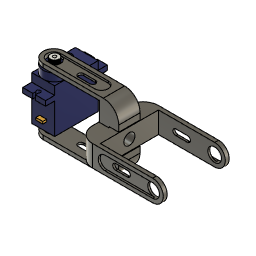
Part_1 v2 (Autodesk Fusion 360 design; units mm, degrees)
Autodesk Fusion 360 part; units mm, degrees
sketch "Left" plane through (0, 0, 0) normal (1, 0, 0) x (0, 0, -1) in component "_Servo-90.427e8e22-afa0-40e2-88ac-6b67eb2e57ee v1"
  line L0 (-21.4055, -22.0984) -> (1.0945, -22.0984)
  line L1 (-21.4055, 4.6016) -> (1.0945, 4.6016)
  line L2 (-21.4055, 0.6016) -> (1.0945, 0.6016)
  line L3 (-21.4055, 0.6016) -> (-21.4055, 4.6016)
  line L4 (5.7945, -22.0984) -> (5.7945, -6.1984)
  line L5 (-26.1055, -6.1984) -> (-26.1055, -3.6984)
  line L6 (-26.1055, -3.6984) -> (-21.4055, -3.6984)
  line L7 (1.0945, -3.6984) -> (5.7945, -3.6984)
  line L8 (-26.1055, -6.1984) -> (-21.4055, -6.1984)
  line L9 (1.0945, -6.1984) -> (5.7945, -6.1984)
  line L10 (1.0945, -22.0984) -> (1.0945, -6.1984)
  line L11 (1.0945, -3.6984) -> (1.0945, 0.6016)
  line L12 (-21.4055, -22.0984) -> (-21.4055, -6.1984)
  line L13 (-21.4055, -3.6984) -> (-21.4055, 0.6016)
  line L14 (-15.5055, 0.6016) -> (-15.5055, 13)
  line L15 (-6.7055, 0.6016) -> (-6.7055, 13)
  line L16 (1.0945, -22.0984) -> (1.0945, -6.1984)
  line L17 (1.0945, -3.6984) -> (1.0945, 13)
  line L18 (5.7945, -3.6984) -> (5.7945, -6.1984)
  dimension "d1" = 22.5
  dimension "d2" = 26.7
  dimension "d3" = 22.7
  dimension "d4" = 4
  dimension "d5" = 22.7
  dimension "d13" = 5.9
  constraint perpendicular L1 L3
  constraint parallel L0 L6
  constraint parallel L0 L8
  constraint parallel L5 L12
  constraint coincident L6.end L12
  constraint coincident L7.start L10
  constraint collinear L6 L7
  constraint collinear L8 L9
  constraint parallel L4 L10
  constraint collinear L10 L11
  constraint collinear L12 L13
  constraint parallel L3 L14
  constraint parallel L14 L16
  constraint collinear L16 L17
  constraint parallel L14 L15
  constraint coincident L2 L15.start
  constraint coincident L2 L14.start
  constraint perpendicular L9 L18
  measures "d1" distance of L0.start L0.end
  measures "d4" distance of L1.start L2.start
  measures "d5" distance of L0.start L2.start
  measures "d13" distance of L3 L14
extrude "Extrude1" add sketch "Left" along normal mid plane 11.8 contours L0 L2 L5 L6 L7 L8 L9 L10 L11 L12 L13 L16 L17 L18 makes body 1 in component "_Servo-90.427e8e22-afa0-40e2-88ac-6b67eb2e57ee v1"
sketch "TOP" plane through (0, 0.6016, 0) normal (0, 1, 0) x (-1, 0, 0) in component "_Servo-90.427e8e22-afa0-40e2-88ac-6b67eb2e57ee v1"
  line L0 (5.9, 21.4055) -> (-5.9, 21.4055)
  line L1 (-5.9, 21.4055) -> (-5.9, -1.0945)
  line L2 (-5.9, -1.0945) -> (5.9, -1.0945)
  line L3 (5.9, -1.0945) -> (5.9, 21.4055)
  circle A0 centre (0, 15.5055) radius 2.3
  circle A1 centre (0, 15.5055) radius 0.85
  line L4 (0, -1.0945) -> (0, 27)
  line L5 (0, 27) -> (0, -1.0945)
  arc A2 (-2.5, 9.2055) -> (2.5, 9.2055) centre (0, 9.2055) ccw
  line L6 (-2.5, 9.2055) -> (-2.5, 10.1613)
  line L7 (2.5, 9.2055) -> (2.5, 10.1613)
  arc A3 (2.5, 10.1613) -> (-2.5, 10.1613) centre (0, 15.5055) ccw
  line L8 (5.9, -5.7945) -> (-5.9, -5.7945)
  line L9 (-0.65, -4.2545) -> (-0.65, -5.7945)
  line L10 (0.65, -4.2545) -> (0.65, -5.7945)
  arc A4 (0.65, -4.2545) -> (-0.65, -4.2545) centre (0, -3.4945) ccw
  line L11 (5.9, 26.1055) -> (-5.9, 26.1055)
  arc A5 (-0.65, 24.5654) -> (0.65, 24.5654) centre (0, 23.8055) ccw
  line L12 (0.65, 24.5654) -> (0.65, 26.1055)
  line L13 (-0.65, 24.5654) -> (-0.65, 26.1055)
  point P0 (0, 15.5055)
  point P1 (0, 6.7055)
  point P2 (0, -1.0945)
  point P3 (5.9, -5.7945)
  point P4 (-5.9, -5.7945)
  point P5 (0, -5.7945)
  point P6 (5.9, 26.1055)
  point P7 (-5.9, 26.1055)
  point P8 (0, 26.1055)
  point P9 (0, 21.4055)
  dimension "d16" = 4.6
  dimension "d17" = 1.7
  dimension "d18" = 11.8
  dimension "d27" = 2
  dimension "d31" = 2
  constraint coincident P0 A0.centre
  constraint concentric A1 A3
  constraint coincident P1 A2
  constraint coincident P2 L4.start
  constraint perpendicular L0 L4
  constraint parallel L4 L6
  constraint parallel L4 L7
  constraint coincident P3 L8.start
  constraint coincident P4 L8.end
  constraint coincident P6 L11.start
  constraint coincident P7 L11.end
  constraint coincident L11 L12.end
  constraint coincident L11 L13.end
  measures "d16" diameter of A0
  measures "d17" diameter of A1
  measures "d18" diameter of A3
  measures "d27" diameter of A4
  measures "d31" diameter of A5
extrude "Extrude2" add sketch "TOP" along normal blind 4 contours A0 L4 L5 A2 L7 A3 | A0 L4 L5 A2 L6 A3 bodies 1 in component "_Servo-90.427e8e22-afa0-40e2-88ac-6b67eb2e57ee v1"
extrude "Extrude3" add sketch "TOP" along normal blind 7.2 separate body contours A0 A1 L4 L5 | A0 A1 L4 L5 makes body 2 in component "_Servo-90.427e8e22-afa0-40e2-88ac-6b67eb2e57ee v1"
extrude "Extrude4" cut sketch "TOP" against normal through all contours L4 L5 L11 A5 L13 | L4 L5 L11 A5 L12 bodies 1 in component "_Servo-90.427e8e22-afa0-40e2-88ac-6b67eb2e57ee v1"
extrude "Extrude5" cut sketch "TOP" against normal through all contours L8 L9 L10 A4 bodies 1 in component "_Servo-90.427e8e22-afa0-40e2-88ac-6b67eb2e57ee v1"
sketch "Front" plane through (0, 0, 21.4055) normal (0, 0, 1) x (1, 0, 0) in component "_Servo-90.427e8e22-afa0-40e2-88ac-6b67eb2e57ee v1"
  line L0 (-5.9, -22.0984) -> (5.9, -22.0984)
  line L1 (5.9, -22.0984) -> (5.9, -6.1984)
  line L2 (5.9, -6.1984) -> (-5.9, -6.1984)
  line L3 (-5.9, -6.1984) -> (-5.9, -22.0984)
  line L4 (-1.8, -17.5984) -> (1.8, -17.5984)
  line L5 (0, -22.0984) -> (0, -6.1984)
  line L6 (1.8, -17.5984) -> (1.8, -16.3984)
  line L7 (-1.8, -17.5984) -> (-1.8, -16.3984)
  line L8 (-1.8, -16.3984) -> (1.8, -16.3984)
extrude "Extrude6" add sketch "Front" along normal blind 2 separate body contours L4 L5 L6 L8 | L4 L5 L7 L8 makes body 3 in component "_Servo-90.427e8e22-afa0-40e2-88ac-6b67eb2e57ee v1"
copy_body "Body->Comp1" bodies 3 removing the originals makes body 4 in component "Prikljiček"
copy_body "Body->Comp2" bodies 2 removing the originals makes body 5 in component "OSovina"
copy_body "Body->Comp3" bodies 1 removing the originals makes body 6 in component "Ohisje"
sketch "Sketch1" plane through (0, 7.8016, 0) normal (0, 1, 0) x (-1, 0, 0) in component "OSovina"
  circle A0 centre (0, 15.5055) radius 0.85
  circle A1 centre (0, 15.5055) radius 2.3
  circle A2 centre (0, 15.5055) radius 2.3
  circle A3 centre (-0.0134, 13.2055) radius 0.125
  dimension "d42" = 0.25
  constraint coincident A2 A3.centre
  measures "d42" diameter of A3
extrude "Extrude1'" cut sketch "Sketch1" against normal up to surface (3.2 mm away) contours A1 A2 A3 | A1 A2 A3 picked at (-0.0101, 13.2473) picked at (-0.0141, 13.1641) bodies 5 in component "OSovina"
pattern_circular "C-Pattern1" count 28 over 360 about axis through (0, 15.4797, 15.5055) along (0, -1, 0) of "Extrude1'" in component "OSovina"
move_body "Move1" bodies 5 to x (1, 0, 0) y (0, 0, 1) z (0, -1, 0) at (0, 5.4071, 22.4039) in component "OSovina"
move_body "Move1'" bodies 6 to x (1, 0, 0) y (0, 0, 1) z (0, -1, 0) at (0, 5.4071, 22.4039) in component "Ohisje"
move_body "Move1''" bodies 4 to x (1, 0, 0) y (0, 0, 1) z (0, -1, 0) at (0, 5.4071, 22.4039) in component "Prikljiček"
sketch "Part_1" plane through (0, 0, 0) normal (0, 0, 1) x (1, 0, 0)
  line L0 (45, -13) -> (20, -13)
  line L1 (20, -2) -> (45, -2)
  line L2 (45, -2) -> (45, -13)
  arc A0 (20, -2) -> (20, -13) centre (20, -7.5) ccw
  circle A1 centre (20, -7.5) radius 3.5
  line L3 (45, -2) -> (59, -2)
  line L4 (59, -13) -> (45, -13)
  line L5 (45, -13) -> (45, -2)
  line L6 (59, -2) -> (59, -13)
  line L7 (20, -4) -> (43, -4)
  line L8 (43, -4) -> (43, -11)
  line L9 (43, -11) -> (20, -11)
  line L10 (40, -6) -> (34, -6)
  line L11 (40, -9) -> (33.9861, -9.0001)
  arc A2 (34, -6) -> (33.9861, -9.0001) centre (33.9861, -7.5) ccw
  arc A3 (40, -9) -> (40, -6) centre (40.068, -7.5) ccw
  constraint horizontal L0
  constraint horizontal L1
  constraint vertical L2
  constraint tangent L0 A0
  constraint horizontal L3
  constraint horizontal L4
  constraint vertical L5
  constraint coincident A1 L7.start
  constraint tangent A1 L7
  constraint horizontal L7
  constraint perpendicular L7 L8
  constraint coincident A1 L9.end
  constraint tangent A1 L9
  constraint perpendicular L8 L9
  constraint perpendicular L8 L10
  constraint tangent L11 A2
extrude "Extrude1''" add sketch "Part_1" along normal blind 30 and the other way blind 4 separate body contours L0 L1 L2 A0 L5 | L2 L3 L4 L5 L6 | A1 L7 L8 L9 makes body 7
sketch "Cut_1" plane through (0, -13, 0) normal (0, -1, 0) x (1, 0, 0)
  line L0 (59, -4) -> (59, 30)
  line L1 (59, 30) -> (20, 30)
  line L2 (20, -4) -> (59, -4)
  line L3 (49, 13) -> (49, 28)
  line L4 (49, 28) -> (13, 28)
  line L5 (13, 28) -> (13, 13)
  line L6 (49, 13) -> (49, -2)
  line L7 (49, -2) -> (13, -2)
  line L8 (13, -2) -> (13, 13)
  line L9 (59, 13) -> (59, 18.5)
  line L10 (59, 13) -> (59, 7.5)
  line L11 (54, 7.5) -> (54, 18.5)
  line L12 (59, 18.5) -> (59, 18.8)
  line L13 (59, 18.8) -> (54, 18.8)
  line L14 (54, 18.8) -> (54, 18.5)
  line L15 (59, 7.5) -> (59, 7.2)
  line L16 (59, 7.2) -> (54, 7.2)
  line L17 (54, 7.2) -> (54, 7.5)
  dimension "d10" = 34
  dimension "d19" = 10
  dimension "d21" = 17
  dimension "d26" = 5.5
  dimension "d28" = 5.5
  dimension "d29" = 5
  dimension "d30" = 11
  dimension "d36" = 0.3
  dimension "d37" = 0.3
  constraint vertical L3
  constraint horizontal L4
  constraint vertical L5
  constraint vertical L6
  constraint horizontal L7
  constraint vertical L8
  constraint parallel L0 L9
  constraint perpendicular L1 L10
  constraint vertical L12
  constraint horizontal L13
  constraint vertical L14
  constraint vertical L15
  constraint horizontal L16
  constraint vertical L17
  measures "d10" distance of L0.start L0.end
  measures "d19" distance of L0 L3.end
  measures "d21" distance of L0.start L9.start
  measures "d26" distance of L9.start L9.end
  measures "d28" distance of L9.start L10.end
  measures "d29" distance of L10.end L11.start
  measures "d30" distance of L11.start L11.end
  measures "d36" distance of L9.end L12.end
  measures "d37" distance of L10.end L15.end
extrude "Extrude2'" cut sketch "Cut_1" against normal blind 16 contours L3 L4 L5 L6 L7 L8 bodies 7
extrude "Extrude3'" cut sketch "Cut_1" against normal blind 16 contours L0 L9 L10 L11 L12 L13 L14 L15 L16 L17 bodies 7
fillet "Fillet1" radius 8 2 edges at (59, -7.5, 30) (59, -7.5, -4) on bodies 7
sketch "Cut_2" plane through (0, 0, 30) normal (0, 0, 1) x (-1, 0, 0)
  line L0 (-51, 13) -> (-51, 2)
  line L1 (-51, 2) -> (-20, 2)
  arc A0 (-20, 2) -> (-20, 13) centre (-20, 7.5) ccw
  line L2 (-20, 13) -> (-51, 13)
  arc A1 (-40, 9) -> (-40, 6) centre (-40.068, 7.5) ccw
  line L3 (-40, 9) -> (-33.9861, 9.0001)
  arc A2 (-34, 6) -> (-33.9861, 9.0001) centre (-33.9861, 7.5) ccw
  line L4 (-34, 6) -> (-40, 6)
  circle A3 centre (-20, 7.5) radius 3.5
  line L5 (-20, 4) -> (-44.5538, 4)
  line L6 (-20, 11) -> (-44.5538, 11)
  arc A4 (-44.5538, 11) -> (-44.5538, 4) centre (-44.5538, 7.5) ccw
  dimension "d51" = 24.5538
  dimension "d53" = 7
  constraint coincident A3 L5.start
  constraint coincident A3 L6.start
  constraint tangent L6 A4
  measures "d51" distance of A0.centre A4.centre
  measures "d53" distance of L5.end L6.end
extrude "Extrude4'" cut sketch "Cut_2" against normal blind 1 contours A3 L5 L6 A4 bodies 7
sketch "Cut_3" plane through (0, 0, -4) normal (0, 0, -1) x (1, 0, 0)
  line L0 (51, 2) -> (51, 13)
  line L1 (51, 13) -> (20, 13)
  arc A0 (20, 13) -> (20, 2) centre (20, 7.5) ccw
  line L2 (20, 2) -> (51, 2)
  circle A1 centre (20, 7.5) radius 3.5
  arc A2 (40, 6) -> (40, 9) centre (40.068, 7.5) ccw
  line L3 (40, 6) -> (34, 6)
  arc A3 (33.9861, 9.0001) -> (34, 6) centre (33.9861, 7.5) ccw
  line L4 (33.9861, 9.0001) -> (40, 9)
  line L5 (20, 11) -> (44.5538, 11)
  line L6 (20, 4) -> (44.5538, 4)
  arc A4 (44.5538, 4) -> (44.5538, 11) centre (44.5538, 7.5) ccw
  dimension "d52" = 24.5538
  dimension "d54" = 7
  constraint coincident A1 L5.start
  constraint tangent L5 A4
  constraint coincident A1 L6.start
  constraint tangent L6 A4
  measures "d52" distance of A0.centre A4.centre
  measures "d54" diameter of A4
extrude "Extrude5'" cut sketch "Cut_3" against normal blind 1 contours A1 L5 L6 A4 bodies 7
sketch "Round_1" plane through (54, 0, 0) normal (1, 0, 0) x (0, 1, 0)
  line L0 (-2, 7.2) -> (-2, 18.8)
  line L1 (-2, 18.8) -> (-13, 18.8)
  line L2 (-13, 18.8) -> (-13, 7.2)
  line L3 (-13, 7.2) -> (-2, 7.2)
  circle A0 centre (-7.5, 13) radius 2.875
  dimension "d57" = 11.6
  dimension "d58" = 5.75
  measures "d57" distance of L1.end L2.end
  measures "d58" diameter of A0
extrude "Extrude6'" cut sketch "Round_1" against normal blind 11 contours A0 bodies 7
move_body "Move4" bodies 7 to x (1, 0, 0) y (0, 1, 0) z (0, 0, 1) at (-4, 0, 0)
move_body "Move5" bodies 7 to x (1, 0, 0) y (0, 1, 0) z (0, 0, 1) at (-16, 0, 0)
copy_body "CopyPasteBodies2" bodies 7 makes body 8
move_body "Move6" bodies 8 to x (-1, -0.000011, -0.000011) y (-0.000011, 0, 1) z (-0.000011, 1, 0) at (67.9862, -20.4995, 20.5002)
component "_Servo-90.427e8e22-afa0-40e2-88ac-6b67eb2e57ee v1" placed x (1, 0, 0) y (0, 1, 0) z (0, 0, 1) at (0, 3, 0)
component "Prikljiček" placed x (1, 0, 0) y (0, 1, 0) z (0, 0, 1) at (0, 0, 0) in component "_Servo-90.427e8e22-afa0-40e2-88ac-6b67eb2e57ee v1"
component "OSovina" placed x (1, 0, 0) y (0, 1, 0) z (0, 0, 1) at (0, 0, 0) in component "_Servo-90.427e8e22-afa0-40e2-88ac-6b67eb2e57ee v1"
component "Ohisje" placed x (1, 0, 0) y (0, 1, 0) z (0, 0, 1) at (0, 0, 0) in component "_Servo-90.427e8e22-afa0-40e2-88ac-6b67eb2e57ee v1"
